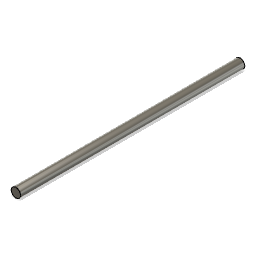
Idea original de arma (Autodesk Fusion 360 archive; units mm, degrees)
design "tubo"
Autodesk Fusion 360 part; units mm, degrees
sketch "Boceto1" plane through (0, 0, 0) normal (0, 0, 1) x (1, 0, 0)
  circle A0 centre (0, 0) radius 5
  dimension "d1" = 10
  constraint coincident A0.centre origin
  measures "d1" diameter of A0
extrude "Extruir1" add sketch "Boceto1" along normal blind 240

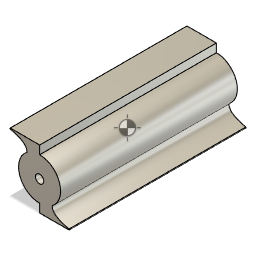
design "Spinner_v6"
Autodesk Fusion 360 part; units mm, degrees
sketch "Boceto1" plane through (0, 0, 0) normal (0, 0, 1) x (1, 0, 0)
  line L0 (0.0132, -25) -> (0.0132, -35)
  line L1 (0.0132, -35) -> (35.0132, -35)
  line L2 (0.1058, 24.9998) -> (0.1058, 34.9998)
  line L3 (0.1058, 34.9998) -> (-34.8942, 34.9998)
  circle A0 centre (0, 0) radius 5
  line L4 (-34.8942, 34.9998) -> (-34.8942, 33.9998)
  line L5 (35.0132, -35) -> (35.0132, -34)
  spline S0 degree 5 poles (-34.8942, 33.9998) (-33.6107, 33.7099) (-31.1097, 33.0928) (-27.5553, 32.0551) (-23.2198, 30.444) (-18.698, 27.933) (-16.1827, 25.3205) (-15.2083, 22.8635) (-15.0273, 20.97) (-15.0541, 19.9593) knots 0 0 0 0 0 0 0.2 0.4 0.6 0.8 1 1 1 1 1 1
  line L6 (-38.6455, 34.8471) -> (-31.1429, 33.1525)
  line L7 (-14.9876, 22.4691) -> (-15.1206, 17.4496)
  spline S1 degree 5 poles (35.0132, -34) (33.7206, -33.7082) (31.2031, -33.0895) (27.6293, -32.0566) (23.2761, -30.4626) (18.7347, -27.9778) (16.1954, -25.3773) (15.1925, -22.9178) (14.9869, -21.0163) (15, -20) knots 0 0 0 0 0 0 0.2 0.4 0.6 0.8 1 1 1 1 1 1
  line L8 (38.7646, -34.8469) -> (31.2618, -33.1531)
  line L9 (14.9677, -22.5104) -> (15.0323, -17.4896)
  arc A1 (-15.0541, 19.9593) -> (0.0132, -25) centre (0, 0) ccw
  arc A2 (15, -20) -> (0.1058, 24.9998) centre (0, 0) ccw
  circle A3 centre (-34.8942, 34.4998) radius 0.5
  circle A4 centre (35.0132, -34.5) radius 0.5
  dimension "d6" = 35
  dimension "d7" = 10
  dimension "d8" = 10
  dimension "d9" = 50
  dimension "d10" = 1
  dimension "d14" = 1
  constraint vertical L0
  constraint perpendicular L0 L1
  constraint coincident S1.end A1
  constraint vertical L2
  constraint perpendicular L2 L3
  constraint concentric A0 A1
  constraint perpendicular L3 L4
  constraint perpendicular L1 L5
  constraint midpoint L4.end L6
  constraint midpoint S0.end L7
  constraint midpoint L5.end L8
  constraint midpoint S1.end L9
  constraint concentric A1 A2
  constraint equal L0 L2
  constraint equal L1 L3
  constraint equal L4 L5
  constraint equal L7 L9
  constraint equal L6 L8
  constraint midpoint L4 A3.centre
  constraint midpoint L5 A4.centre
  constraint equal A3 A4
  measures "d6" distance of L2.end L3.end
  measures "d7" distance of L2.start L2.end
  measures "d8" diameter of A0
  measures "d9" diameter of A1
  measures "d10" distance of L1.end L5.end
  measures "d14" diameter of A4
extrude "Extruir4" add sketch "Boceto1" along normal blind 210
move_body "Desplazar1" bodies 1 to x (1, 0, 0) y (0, 1, 0) z (0, 0, 1) at (0, 0, -105)
equation "d14 = d10"
named bodies: "ArmaFinalsinFilo"

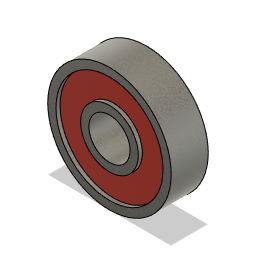
design "Rodamiento Básico"
Autodesk Fusion 360 part; units mm, degrees
sketch "Boceto1" plane through (0, 0, 0) normal (0, 0, 1) x (1, 0, 0)
  circle A0 centre (0, 0) radius 5
  circle A1 centre (0, 0) radius 15
  circle A2 centre (0, 0) radius 13
  circle A3 centre (0, 0) radius 7
  dimension "d1" = 10
  dimension "d2" = 30
  dimension "d3" = 26
  dimension "d4" = 14
  constraint coincident A0.centre A1.centre
  constraint concentric A1 A2
  constraint concentric A0 A3
  measures "d1" diameter of A0
  measures "d2" diameter of A1
  measures "d3" diameter of A2
  measures "d4" diameter of A3
extrude "Extruir1" add sketch "Boceto1" along normal blind 9 makes body 1 at (14.9255, -1.4935, 3) makes body 2 at (6.9913, -0.3489, 6)
extrude "Extruir2" add sketch "Boceto1" along normal blind 7 separate body contours A2 makes body 3
move_body "Desplazar1" bodies 3 to x (1, 0, 0) y (0, 1, 0) z (0, 0, 1) at (0, 0, 1)
combine "Combinar1" operation add target body 2 tool bodies 3 1
named bodies: "Rodamiento"
